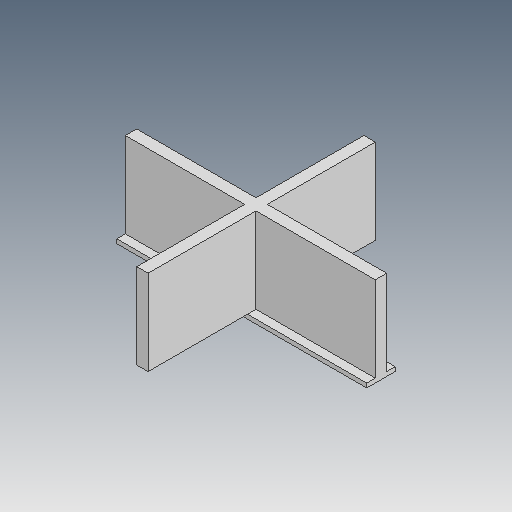
# Autodesk Inventor part: halfdrawerdivider
Saved by Autodesk Inventor 2025.2 (Build 292293000, 293)
## iProperties
Created: 2025-02-25
Part Number: halfdrawerdivider
Material: Generic
Document SubType Name: Modeling
Designer: email
Density: 1 g/cm^3
Appearance: Default
Author: email
Autodesk Inventor part; units mm, degrees
ref_plane "YZ Plane" through (0, 0, 0) normal (1, 0, 0) x (0, 1, 0)
ref_plane "XZ Plane" through (0, 0, 0) normal (0, 1, 0) x (-1, 0, 0)
ref_plane "XY Plane" through (0, 0, 0) normal (0, 0, 1) x (1, 0, 0)
sketch "Sketch2" plane through (0, 0, 0) normal (0, 1, 0) x (-1, 0, 0)
  line L0 (2, -40) -> (-2, -40)
  line L1 (-2, -40) -> (-2, 40)
  line L2 (-2, 40) -> (2, 40)
  line L3 (2, 40) -> (2, -40)
  line L4 (44, -2) -> (-44, -2)
  line L5 (-44, -2) -> (-44, 2)
  line L6 (-44, 2) -> (44, 2)
  line L7 (44, 2) -> (44, -2)
  line L8 (44, 5) -> (-44, 5)
  line L9 (-44, 5) -> (-44, -5)
  line L10 (-44, -5) -> (44, -5)
  line L11 (44, -5) -> (44, 5)
  point P0 (0, 0)
  point P1 (0, -40)
  point P2 (-44, 0)
  point P3 (0, -2)
  point P4 (-2, 0)
  point P5 (2, 2)
  point P6 (-2, 2)
  point P7 (-2, -2)
  point P8 (2, -2)
  point P9 (44, 0)
  dimension "d0" = 4
  dimension "d1" = 4
  dimension "d2" = 80
  dimension "d3" = 88
  dimension "d6" = 10
  constraints: 24 end point, 6 parallel, 5 midpoint, 3 horizontal, 3 horizontal alignment, 3 perpendicular, 2 collinear, 2 vertical alignment
  measures "d0" distance between parallel lines of L1 L3
  measures "d1" distance between parallel lines of L6 L4
  measures "d2" distance of L0.end L1.end
  measures "d3" distance of L5.end L6.end
  measures "d6" distance between parallel lines of L8 L10
extrude "Extrusion1" add sketch "Sketch2" along normal blind 30 contours L0 L1 L10 L3 | L10 L1 L4 L3 | L4 L1 L6 L3 | L3 L6 L7 L4 | L4 L5 L6 L1 | L6 L1 L8 L3 | L8 L1 L2 L3
extrude "Extrusion2" add sketch "Sketch2" against normal blind 1.5 contours L10 L1 L4 L3 | L3 L4 L11 L10 | L10 L9 L4 L1 | L4 L1 L6 L3 | L3 L6 L7 L4 | L4 L5 L6 L1 | L6 L1 L8 L3 | L3 L8 L11 L6 | L6 L9 L8 L1
body "Solid1"
